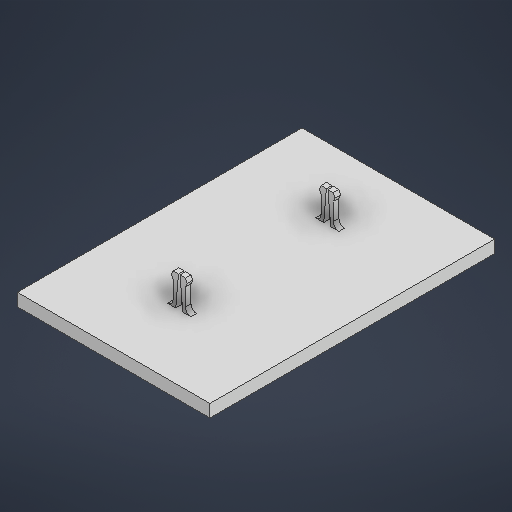
# Autodesk Inventor part: Bolt Slot Covers
Saved by Autodesk Inventor 2026.2 (Build 302298000, 298)
## iProperties
Created: 2026-05-27
Part Number: Bolt Slot Covers
Material: Generic
Document SubType Name: Modeling
Designer: mayhe
Density: 1 g/cm^3
Appearance: Default
Author: mayhe
Autodesk Inventor part; units mm, degrees
ref_plane "YZ Plane" through (0, 0, 0) normal (1, 0, 0) x (0, 1, 0)
ref_plane "XZ Plane" through (0, 0, 0) normal (0, 1, 0) x (-1, 0, 0)
ref_plane "XY Plane" through (0, 0, 0) normal (0, 0, 1) x (1, 0, 0)
sketch "Sketch1" plane through (0, 0, 0) normal (0, 1, 0) x (-1, 0, 0)
  line L0 (34.5, 51) -> (-34.5, 51)
  line L1 (-34.5, 51) -> (-34.5, -51)
  line L2 (-34.5, -51) -> (34.5, -51)
  line L3 (34.5, -51) -> (34.5, 51)
  line L4 (34.5, 51) -> (-34.5, -51) construction
  line L5 (-34.5, 51) -> (34.5, -51) construction
  point P0 (0, 0)
  dimension "d0" = 69
  dimension "d1" = 102
  constraints: 12 end point, 2 midpoint, 2 parallel, 1 horizontal, 1 perpendicular
  measures "d0" distance of L2.end L1.end
  measures "d1" distance of L1.end L0.end
extrude "Extrusion1" add sketch "Sketch1" along normal mid plane 5
sketch "Sketch3" plane through (0, 2.5, 0) normal (0, 1, 0) x (1, 0, 0)
  line L0 (0, 26.5) -> (0, -26.5)
  line L1 (-2.2, 27.5) -> (2.2, 27.5)
  line L2 (2.2, 27.5) -> (2.2, 25.5)
  line L3 (2.2, 25.5) -> (-2.2, 25.5)
  line L4 (-2.2, 25.5) -> (-2.2, 27.5)
  line L5 (-2.2, 27.5) -> (2.2, 25.5) construction
  line L6 (2.2, 27.5) -> (-2.2, 25.5) construction
  line L7 (-1.25, 27.5) -> (1.25, 27.5)
  line L8 (1.25, 27.5) -> (1.25, 25.5)
  line L9 (1.25, 25.5) -> (-1.25, 25.5)
  line L10 (-1.25, 25.5) -> (-1.25, 27.5)
  line L11 (-1.25, 27.5) -> (1.25, 25.5) construction
  line L12 (1.25, 27.5) -> (-1.25, 25.5) construction
  point P0 (0, 0)
  point P1 (1.25, 27.5)
  point P2 (-1.25, 25.5)
  point P3 (-1.25, 27.5)
  dimension "d13" = 53
  dimension "d14" = 4.4
  dimension "d15" = 2
  dimension "d18" = 2.5
  constraints: 26 end point, 5 midpoint, 4 parallel, 2 horizontal, 2 perpendicular, 1 point on line, 1 vertical
  measures "d13" distance of L0.start L0.end
  measures "d14" distance of L2.end L3.end
  measures "d15" distance between parallel lines of L3 L1
  measures "d18" distance of L8.end L9.end
extrude "Extrusion3" add sketch "Sketch3" along normal blind 11 contours L1 L2 L3 L8
sketch "Sketch4" plane through (2.2, 2.5, -27.5) normal (0, 0, -1) x (-1, 0, 0)
  line L0 (0, 0) -> (0, 11) projected
  line L1 (0, 11) -> (-0.6339, 9.6405)
  line L2 (0, 11) -> (1.5, 11) construction
  line L3 (-0.6339, 9.6405) -> (0, 8.2811)
  point P0 (2.2, -2.5)
  point P1 (0, 8.2811)
  dimension "d19" = 1.5
  dimension "d20" = 115
  dimension "d21" = 1.5
  constraints: 6 end point, 1 equal length, 1 horizontal
  measures "d19" distance of L0.end L1.end
  measures "d20" angle of L1 L2
  measures "d21" distance of L1.end L3.end
extrude "Extrusion4" add sketch "Sketch4" against normal up to surface (2 mm away)
fillet "Fillet1" radius 2 1 edges at (2.2, 2.5, -26.5)
draft "FaceDraft1" angle -5 pull direction (0, 1, 0) faces at (1.25, 6.1667, -26.8333) fixed edges at (1.25, 2.5, -26.5)
mirror "Mirror1" about plane through (0, 0, 0) normal (1, 0, 0) of "Extrusion4", "Extrusion3", "FaceDraft1", "Fillet1"
mirror "Mirror2" about plane through (0, 0, 0) normal (0, 0, 1) of "Extrusion4", "Extrusion3", "FaceDraft1", "Fillet1", "Mirror1"
chamfer "Chamfer2" distance 0.5 angle 45 4 edges at (0, -2.5, 51) (34.5, -2.5, 0) (-34.5, -2.5, 0) (0, -2.5, -51)
sketch "Sketch5" plane through (0, -2.5, 0) normal (0, -1, 0) x (1, 0, 0)
  line L0 (-43.2011, -30.2935) -> (-43.2011, 28.7129) construction
  line L1 (-43.2011, 28.7129) -> (40.8303, 28.7129) construction
  line L2 (40.8303, 28.7129) -> (40.8303, -30.2935) construction
  line L3 (40.8303, -30.2935) -> (-43.2011, -30.2935) construction
  spline S0 degree 2 poles (-3.5733, -17.3493) (-3.5733, -18.0112) (-3.8499, -18.9399) (-4.0475, -19.35) knots 0 0 0 1 2 2 2
  line L4 (-4.0475, -19.35) -> (-5.0652, -19.35)
  line L5 (-5.0652, -19.35) -> (-5.0652, -19.2907)
  spline S1 degree 2 poles (-5.0652, -19.2907) (-4.6897, -18.8905) (-4.2748, -17.8778) (-4.2748, -17.4085) knots 0 0 0 1 2 2 2
  spline S2 degree 2 poles (-4.2748, -17.4085) (-4.2748, -16.7367) (-4.833, -16.05) (-5.2924, -16.05) knots 0 0 0 1 2 2 2
  spline S3 degree 2 poles (-5.2924, -16.05) (-5.658, -16.05) (-6.1125, -16.4106) (-6.2261, -16.8009) knots 0 0 0 1 2 2 2
  spline S4 degree 2 poles (-6.2261, -16.8009) (-6.3051, -17.0825) (-6.4138, -17.5518) (-6.5027, -17.9025) knots 0 0 0 1 2 2 2
  spline S5 degree 2 poles (-6.5027, -17.9025) (-6.5867, -18.2187) (-6.8386, -18.7176) (-7.0412, -18.9103) knots 0 0 0 1 2 2 2
  spline S6 degree 2 poles (-7.0412, -18.9103) (-7.2437, -19.098) (-7.7871, -19.3055) (-8.1428, -19.3055) knots 0 0 0 1 2 2 2
  spline S7 degree 2 poles (-8.1428, -19.3055) (-8.8838, -19.3055) (-9.8866, -18.1495) (-9.8866, -17.2554) knots 0 0 0 1 2 2 2
  spline S8 degree 2 poles (-9.8866, -17.2554) (-9.8866, -16.7416) (-9.6841, -15.8327) (-9.4914, -15.4424) knots 0 0 0 1 2 2 2
  line L6 (-9.4914, -15.4424) -> (-8.5232, -15.4424)
  line L7 (-8.5232, -15.4424) -> (-8.5232, -15.5017)
  spline S9 degree 2 poles (-8.5232, -15.5017) (-8.79, -15.7931) (-9.1852, -16.7021) (-9.1852, -17.2011) knots 0 0 0 1 2 2 2
  spline S10 degree 2 poles (-9.1852, -17.2011) (-9.1852, -17.7642) (-8.6566, -18.4608) (-8.2268, -18.4608) knots 0 0 0 1 2 2 2
  spline S11 degree 2 poles (-8.2268, -18.4608) (-7.8415, -18.4608) (-7.382, -18.0507) (-7.2783, -17.6654) knots 0 0 0 1 2 2 2
  spline S12 degree 2 poles (-7.2783, -17.6654) (-7.2091, -17.4085) (-7.0313, -16.6626) (-6.9572, -16.4156) knots 0 0 0 1 2 2 2
  spline S13 degree 2 poles (-6.9572, -16.4156) (-6.7645, -15.7882) (-5.989, -15.2053) (-5.4209, -15.2053) knots 0 0 0 1 2 2 2
  spline S14 degree 2 poles (-5.4209, -15.2053) (-5.0602, -15.2053) (-4.3686, -15.4967) (-4.1266, -15.7586) knots 0 0 0 1 2 2 2
  spline S15 degree 2 poles (-4.1266, -15.7586) (-3.8598, -16.05) (-3.5733, -16.791) (-3.5733, -17.3493) knots 0 0 0 1 2 2 2
  line L8 (-3.682, -13.6541) -> (-3.682, -14.4248)
  line L9 (-3.682, -14.4248) -> (-10.0497, -14.4248)
  line L10 (-10.0497, -14.4248) -> (-10.0497, -13.6541)
  line L11 (-10.0497, -13.6541) -> (-3.682, -13.6541)
  spline S16 degree 2 poles (-5.9692, -8.7635) (-4.8132, -8.7635) (-3.5535, -9.875) (-3.5535, -10.8037) knots 0 0 0 1 2 2 2
  spline S17 degree 2 poles (-3.5535, -10.8037) (-3.5535, -11.7571) (-4.8527, -12.8489) (-5.9692, -12.8489) knots 0 0 0 1 2 2 2
  spline S18 degree 2 poles (-5.9692, -12.8489) (-7.1153, -12.8489) (-8.3849, -11.7226) (-8.3849, -10.8037) knots 0 0 0 1 2 2 2
  spline S19 degree 2 poles (-8.3849, -10.8037) (-8.3849, -9.875) (-7.1202, -8.7635) (-5.9692, -8.7635) knots 0 0 0 1 2 2 2
  spline S20 degree 2 poles (-5.9692, -9.5588) (-6.8584, -9.5588) (-7.7229, -10.206) (-7.7229, -10.8037) knots 0 0 0 1 2 2 2
  spline S21 degree 2 poles (-7.7229, -10.8037) (-7.7229, -11.4015) (-6.8584, -12.0535) (-5.9692, -12.0535) knots 0 0 0 1 2 2 2
  spline S22 degree 2 poles (-5.9692, -12.0535) (-5.1047, -12.0535) (-4.2155, -11.4015) (-4.2155, -10.8037) knots 0 0 0 1 2 2 2
  spline S23 degree 2 poles (-4.2155, -10.8037) (-4.2155, -10.2109) (-5.0899, -9.5588) (-5.9692, -9.5588) knots 0 0 0 1 2 2 2
  spline S24 degree 2 poles (-3.593, -6.5899) (-3.593, -7.2172) (-4.3093, -7.9237) (-5.0849, -7.9237) knots 0 0 0 1 2 2 2
  line L12 (-5.0849, -7.9237) -> (-7.6192, -7.9237)
  line L13 (-7.6192, -7.9237) -> (-7.6192, -8.4424)
  line L14 (-7.6192, -8.4424) -> (-8.2564, -8.4424)
  line L15 (-8.2564, -8.4424) -> (-8.2564, -7.9237)
  line L16 (-8.2564, -7.9237) -> (-9.5705, -7.9237)
  line L17 (-9.5705, -7.9237) -> (-9.5705, -7.153)
  line L18 (-9.5705, -7.153) -> (-8.2564, -7.153)
  line L19 (-8.2564, -7.153) -> (-8.2564, -5.7352)
  line L20 (-8.2564, -5.7352) -> (-7.6192, -5.7352)
  line L21 (-7.6192, -5.7352) -> (-7.6192, -7.153)
  line L22 (-7.6192, -7.153) -> (-5.4406, -7.153)
  spline S25 degree 2 poles (-5.4406, -7.153) (-5.0948, -7.153) (-4.7144, -7.1283) (-4.5514, -7.0443) knots 0 0 0 1 2 2 2
  spline S26 degree 2 poles (-4.5514, -7.0443) (-4.4081, -6.9752) (-4.2649, -6.664) (-4.2649, -6.3972) knots 0 0 0 1 2 2 2
  spline S27 degree 2 poles (-4.2649, -6.3972) (-4.2649, -6.2095) (-4.3785, -5.8587) (-4.4131, -5.7797) knots 0 0 0 1 2 2 2
  line L23 (-4.4131, -5.7797) -> (-4.4131, -5.7352)
  line L24 (-4.4131, -5.7352) -> (-3.7215, -5.7352)
  spline S28 degree 2 poles (-3.7215, -5.7352) (-3.6622, -5.9526) (-3.593, -6.3972) (-3.593, -6.5899) knots 0 0 0 1 2 2 2
  spline S29 degree 2 poles (-3.5733, -0.1085) (-3.5733, -0.7013) (-3.9734, -1.7042) (-4.3736, -2.0697) knots 0 0 0 1 2 2 2
  spline S30 degree 2 poles (-4.3736, -2.0697) (-4.7688, -2.4353) (-5.9544, -2.8354) (-6.725, -2.8354) knots 0 0 0 1 2 2 2
  spline S31 degree 2 poles (-6.725, -2.8354) (-7.4907, -2.8354) (-8.6269, -2.4452) (-9.0468, -2.0747) knots 0 0 0 1 2 2 2
  spline S32 degree 2 poles (-9.0468, -2.0747) (-9.4569, -1.7091) (-9.8866, -0.7112) (-9.8866, -0.0937) knots 0 0 0 1 2 2 2
  spline S33 degree 2 poles (-9.8866, -0.0937) (-9.8866, 0.2126) (-9.7977, 0.751) (-9.7286, 0.9783) knots 0 0 0 1 2 2 2
  spline S34 degree 2 poles (-9.7286, 0.9783) (-9.6643, 1.1759) (-9.4816, 1.5859) (-9.3729, 1.7884) knots 0 0 0 1 2 2 2
  line L25 (-9.3729, 1.7884) -> (-8.3948, 1.7884)
  line L26 (-8.3948, 1.7884) -> (-8.3948, 1.7242)
  spline S35 degree 2 poles (-8.3948, 1.7242) (-8.4936, 1.6155) (-8.7702, 1.2796) (-8.9036, 1.0375) knots 0 0 0 1 2 2 2
  spline S36 degree 2 poles (-8.9036, 1.0375) (-9.032, 0.8054) (-9.195, 0.257) (-9.195, -0.0987) knots 0 0 0 1 2 2 2
  spline S37 degree 2 poles (-9.195, -0.0987) (-9.195, -0.4889) (-8.8739, -1.1855) (-8.5677, -1.4473) knots 0 0 0 1 2 2 2
  spline S38 degree 2 poles (-8.5677, -1.4473) (-8.2564, -1.7042) (-7.3129, -1.9907) (-6.725, -1.9907) knots 0 0 0 1 2 2 2
  spline S39 degree 2 poles (-6.725, -1.9907) (-6.0976, -1.9907) (-5.1936, -1.6894) (-4.8824, -1.4275) knots 0 0 0 1 2 2 2
  spline S40 degree 2 poles (-4.8824, -1.4275) (-4.581, -1.1706) (-4.2748, -0.484) (-4.2748, -0.0987) knots 0 0 0 1 2 2 2
  spline S41 degree 2 poles (-4.2748, -0.0987) (-4.2748, 0.2521) (-4.4477, 0.8498) (-4.5761, 1.082) knots 0 0 0 1 2 2 2
  spline S42 degree 2 poles (-4.5761, 1.082) (-4.7045, 1.3043) (-4.9713, 1.6353) (-5.0652, 1.7292) knots 0 0 0 1 2 2 2
  line L27 (-5.0652, 1.7292) -> (-5.0652, 1.7884)
  line L28 (-5.0652, 1.7884) -> (-4.0969, 1.7884)
  spline S43 degree 2 poles (-4.0969, 1.7884) (-4.0031, 1.5859) (-3.8302, 1.2302) (-3.7511, 0.9783) knots 0 0 0 1 2 2 2
  spline S44 degree 2 poles (-3.7511, 0.9783) (-3.6622, 0.7115) (-3.5733, 0.257) (-3.5733, -0.1085) knots 0 0 0 1 2 2 2
  spline S45 degree 2 poles (-5.9692, 6.2443) (-4.8132, 6.2443) (-3.5535, 5.1328) (-3.5535, 4.2041) knots 0 0 0 1 2 2 2
  spline S46 degree 2 poles (-3.5535, 4.2041) (-3.5535, 3.2507) (-4.8527, 2.1589) (-5.9692, 2.1589) knots 0 0 0 1 2 2 2
  spline S47 degree 2 poles (-5.9692, 2.1589) (-7.1153, 2.1589) (-8.3849, 3.2853) (-8.3849, 4.2041) knots 0 0 0 1 2 2 2
  spline S48 degree 2 poles (-8.3849, 4.2041) (-8.3849, 5.1328) (-7.1202, 6.2443) (-5.9692, 6.2443) knots 0 0 0 1 2 2 2
  spline S49 degree 2 poles (-5.9692, 5.449) (-6.8584, 5.449) (-7.7229, 4.8019) (-7.7229, 4.2041) knots 0 0 0 1 2 2 2
  spline S50 degree 2 poles (-7.7229, 4.2041) (-7.7229, 3.6064) (-6.8584, 2.9543) (-5.9692, 2.9543) knots 0 0 0 1 2 2 2
  spline S51 degree 2 poles (-5.9692, 2.9543) (-5.1047, 2.9543) (-4.2155, 3.6064) (-4.2155, 4.2041) knots 0 0 0 1 2 2 2
  spline S52 degree 2 poles (-4.2155, 4.2041) (-4.2155, 4.7969) (-5.0899, 5.449) (-5.9692, 5.449) knots 0 0 0 1 2 2 2
  line L29 (-8.2564, 10.6262) -> (-3.682, 8.9021)
  line L30 (-3.682, 8.9021) -> (-3.682, 8.2105)
  line L31 (-3.682, 8.2105) -> (-8.2564, 6.5012)
  line L32 (-8.2564, 6.5012) -> (-8.2564, 7.3361)
  line L33 (-8.2564, 7.3361) -> (-4.7342, 8.5859)
  line L34 (-4.7342, 8.5859) -> (-8.2564, 9.8259)
  line L35 (-8.2564, 9.8259) -> (-8.2564, 10.6262)
  spline S53 degree 2 poles (-3.5782, 13.195) (-3.5782, 12.0983) (-4.8083, 10.8929) (-5.9445, 10.8929) knots 0 0 0 1 2 2 2
  spline S54 degree 2 poles (-5.9445, 10.8929) (-7.0609, 10.8929) (-8.3849, 12.0637) (-8.3849, 13.0072) knots 0 0 0 1 2 2 2
  spline S55 degree 2 poles (-8.3849, 13.0072) (-8.3849, 13.4321) (-8.1379, 14.0891) (-7.876, 14.3312) knots 0 0 0 1 2 2 2
  spline S56 degree 2 poles (-7.876, 14.3312) (-7.6142, 14.5782) (-6.8584, 14.84) (-6.3101, 14.84) knots 0 0 0 1 2 2 2
  line L36 (-6.3101, 14.84) -> (-5.8902, 14.84)
  line L37 (-5.8902, 14.84) -> (-5.8902, 11.6734)
  spline S57 degree 2 poles (-5.8902, 11.6734) (-5.0948, 11.6734) (-4.2501, 12.4737) (-4.2501, 13.1851) knots 0 0 0 1 2 2 2
  spline S58 degree 2 poles (-4.2501, 13.1851) (-4.2501, 13.437) (-4.3637, 13.9261) (-4.4526, 14.1237) knots 0 0 0 1 2 2 2
  spline S59 degree 2 poles (-4.4526, 14.1237) (-4.5514, 14.3312) (-4.7243, 14.6177) (-4.8033, 14.7116) knots 0 0 0 1 2 2 2
  line L38 (-4.8033, 14.7116) -> (-4.8033, 14.756)
  line L39 (-4.8033, 14.756) -> (-3.9635, 14.756)
  spline S60 degree 2 poles (-3.9635, 14.756) (-3.9092, 14.6226) (-3.7511, 14.2176) (-3.7067, 14.0595) knots 0 0 0 1 2 2 2
  spline S61 degree 2 poles (-3.7067, 14.0595) (-3.6424, 13.8372) (-3.5782, 13.4716) (-3.5782, 13.195) knots 0 0 0 1 2 2 2
  spline S62 degree 2 poles (-6.478, 14.0891) (-6.7892, 14.0792) (-7.2437, 13.9508) (-7.3969, 13.8273) knots 0 0 0 1 2 2 2
  spline S63 degree 2 poles (-7.3969, 13.8273) (-7.5698, 13.6939) (-7.7525, 13.274) (-7.7525, 12.9628) knots 0 0 0 1 2 2 2
  spline S64 degree 2 poles (-7.7525, 12.9628) (-7.7525, 12.6565) (-7.5698, 12.2267) (-7.3919, 12.0489) knots 0 0 0 1 2 2 2
  spline S65 degree 2 poles (-7.3919, 12.0489) (-7.2091, 11.876) (-6.7695, 11.6981) (-6.478, 11.6734) knots 0 0 0 1 2 2 2
  line L40 (-6.478, 11.6734) -> (-6.478, 14.0891)
  line L41 (-7.4314, 18.0461) -> (-7.4314, 18.0066)
  spline S66 degree 2 poles (-7.4314, 18.0066) (-7.4561, 17.9176) (-7.466, 17.725) (-7.466, 17.5916) knots 0 0 0 1 2 2 2
  spline S67 degree 2 poles (-7.466, 17.5916) (-7.466, 17.2804) (-7.1943, 16.6678) (-6.9276, 16.3912) knots 0 0 0 1 2 2 2
  line L42 (-6.9276, 16.3912) -> (-3.682, 16.3912)
  line L43 (-3.682, 16.3912) -> (-3.682, 15.6205)
  line L44 (-3.682, 15.6205) -> (-8.2564, 15.6205)
  line L45 (-8.2564, 15.6205) -> (-8.2564, 16.3912)
  line L46 (-8.2564, 16.3912) -> (-7.5747, 16.3912)
  spline S68 degree 2 poles (-7.5747, 16.3912) (-7.9502, 16.8111) (-8.2564, 17.4385) (-8.2564, 17.7349) knots 0 0 0 1 2 2 2
  spline S69 degree 2 poles (-8.2564, 17.7349) (-8.2564, 17.8534) (-8.2466, 17.972) (-8.2317, 18.0461) knots 0 0 0 1 2 2 2
  line L47 (-8.2317, 18.0461) -> (-7.4314, 18.0461)
  spline S70 degree 2 poles (4.4184, -15.8672) (4.8581, -15.8672) (5.609, -16.1488) (5.8856, -16.4057) knots 0 0 0 1 2 2 2
  spline S71 degree 2 poles (5.8856, -16.4057) (6.1623, -16.6626) (6.4834, -17.4283) (6.4834, -17.9025) knots 0 0 0 1 2 2 2
  spline S72 degree 2 poles (6.4834, -17.9025) (6.4834, -18.3373) (6.2907, -19.1869) (6.1376, -19.4982) knots 0 0 0 1 2 2 2
  line L48 (6.1376, -19.4982) -> (5.2731, -19.4982)
  line L49 (5.2731, -19.4982) -> (5.2731, -19.4389)
  spline S73 degree 2 poles (5.2731, -19.4389) (5.3422, -19.345) (5.5201, -18.9943) (5.5991, -18.7819) knots 0 0 0 1 2 2 2
  spline S74 degree 2 poles (5.5991, -18.7819) (5.6831, -18.5398) (5.777, -18.1397) (5.777, -17.8877) knots 0 0 0 1 2 2 2
  spline S75 degree 2 poles (5.777, -17.8877) (5.777, -17.6407) (5.5991, -17.1764) (5.4065, -17.0084) knots 0 0 0 1 2 2 2
  spline S76 degree 2 poles (5.4065, -17.0084) (5.2237, -16.8552) (4.7396, -16.6972) (4.4135, -16.6972) knots 0 0 0 1 2 2 2
  spline S77 degree 2 poles (4.4135, -16.6972) (4.0875, -16.6972) (3.6725, -16.875) (3.5342, -17.043) knots 0 0 0 1 2 2 2
  spline S78 degree 2 poles (3.5342, -17.043) (3.381, -17.2159) (3.2526, -17.7296) (3.2526, -18.0409) knots 0 0 0 1 2 2 2
  spline S79 degree 2 poles (3.2526, -18.0409) (3.2526, -18.3768) (3.3563, -19.0437) (3.4008, -19.2462) knots 0 0 0 1 2 2 2
  line L50 (3.4008, -19.2462) -> (0.2589, -19.2462)
  line L51 (0.2589, -19.2462) -> (0.2589, -15.9018)
  line L52 (0.2589, -15.9018) -> (0.9752, -15.9018)
  line L53 (0.9752, -15.9018) -> (0.9752, -18.4608)
  line L54 (0.9752, -18.4608) -> (2.6005, -18.4608)
  spline S80 degree 2 poles (2.6005, -18.4608) (2.5808, -18.3126) (2.5659, -18.026) (2.5659, -17.9075) knots 0 0 0 1 2 2 2
  spline S81 degree 2 poles (2.5659, -17.9075) (2.5659, -17.4382) (2.7191, -16.791) (2.9463, -16.4946) knots 0 0 0 1 2 2 2
  spline S82 degree 2 poles (2.9463, -16.4946) (3.1736, -16.1933) (3.8652, -15.8672) (4.4184, -15.8672) knots 0 0 0 1 2 2 2
  line L55 (-0.0128, -12.4537) -> (7.6789, -14.8397)
  line L56 (7.6789, -14.8397) -> (7.6789, -15.5313)
  line L57 (7.6789, -15.5313) -> (-0.0128, -13.1552)
  line L58 (-0.0128, -13.1552) -> (-0.0128, -12.4537)
  line L59 (6.3549, -8.0225) -> (6.3549, -11.7818)
  line L60 (6.3549, -11.7818) -> (5.4904, -11.7818)
  spline S83 degree 2 poles (5.4904, -11.7818) (5.1101, -11.3768) (4.4036, -10.6555) (4.0232, -10.3097) knots 0 0 0 1 2 2 2
  spline S84 degree 2 poles (4.0232, -10.3097) (3.2575, -9.6132) (2.3387, -9.1043) (1.8496, -9.1043) knots 0 0 0 1 2 2 2
  spline S85 degree 2 poles (1.8496, -9.1043) (1.5928, -9.1043) (1.2074, -9.2624) (1.0839, -9.4057) knots 0 0 0 1 2 2 2
  spline S86 degree 2 poles (1.0839, -9.4057) (0.9604, -9.5489) (0.8369, -9.9244) (0.8369, -10.1516) knots 0 0 0 1 2 2 2
  spline S87 degree 2 poles (0.8369, -10.1516) (0.8369, -10.369) (0.9456, -10.8136) (1.0296, -11.0161) knots 0 0 0 1 2 2 2
  spline S88 degree 2 poles (1.0296, -11.0161) (1.0987, -11.189) (1.2963, -11.5101) (1.3655, -11.6089) knots 0 0 0 1 2 2 2
  line L61 (1.3655, -11.6089) -> (1.3655, -11.6534)
  line L62 (1.3655, -11.6534) -> (0.4961, -11.6534)
  spline S89 degree 2 poles (0.4961, -11.6534) (0.3726, -11.4015) (0.1305, -10.4974) (0.1305, -10.0923) knots 0 0 0 1 2 2 2
  spline S90 degree 2 poles (0.1305, -10.0923) (0.1305, -9.2377) (1.0345, -8.2744) (1.8052, -8.2744) knots 0 0 0 1 2 2 2
  spline S91 degree 2 poles (1.8052, -8.2744) (2.1658, -8.2744) (2.7685, -8.4424) (3.0254, -8.5906) knots 0 0 0 1 2 2 2
  spline S92 degree 2 poles (3.0254, -8.5906) (3.2921, -8.7388) (3.8158, -9.1686) (4.0677, -9.4057) knots 0 0 0 1 2 2 2
  spline S93 degree 2 poles (4.0677, -9.4057) (4.4876, -9.791) (5.3867, -10.7345) (5.6485, -11.0161) knots 0 0 0 1 2 2 2
  line L63 (5.6485, -11.0161) -> (5.6485, -8.0225)
  line L64 (5.6485, -8.0225) -> (6.3549, -8.0225)
  spline S94 degree 2 poles (6.4933, -5.3647) (6.4933, -5.8192) (6.2216, -6.5652) (5.9696, -6.827) knots 0 0 0 1 2 2 2
  spline S95 degree 2 poles (5.9696, -6.827) (5.7226, -7.0839) (5.0508, -7.3506) (4.6704, -7.3506) knots 0 0 0 1 2 2 2
  spline S96 degree 2 poles (4.6704, -7.3506) (4.1764, -7.3506) (3.3465, -6.822) (3.0995, -6.3182) knots 0 0 0 1 2 2 2
  line L65 (3.0995, -6.3182) -> (3.0748, -6.3182)
  spline S97 degree 2 poles (3.0748, -6.3182) (2.8129, -6.7677) (2.1905, -7.2024) (1.7261, -7.2024) knots 0 0 0 1 2 2 2
  spline S98 degree 2 poles (1.7261, -7.2024) (1.0395, -7.2024) (0.1206, -6.165) (0.1206, -5.3647) knots 0 0 0 1 2 2 2
  spline S99 degree 2 poles (0.1206, -5.3647) (0.1206, -4.5348) (0.9901, -3.532) (1.6718, -3.532) knots 0 0 0 1 2 2 2
  spline S100 degree 2 poles (1.6718, -3.532) (2.0818, -3.532) (2.8821, -4.0112) (3.1093, -4.4607) knots 0 0 0 1 2 2 2
  line L66 (3.1093, -4.4607) -> (3.134, -4.4607)
  spline S101 degree 2 poles (3.134, -4.4607) (3.381, -3.9272) (4.0924, -3.3788) (4.6556, -3.3788) knots 0 0 0 1 2 2 2
  spline S102 degree 2 poles (4.6556, -3.3788) (5.4361, -3.3788) (6.4933, -4.515) (6.4933, -5.3647) knots 0 0 0 1 2 2 2
  spline S103 degree 2 poles (4.7346, -4.2186) (4.3592, -4.2186) (3.9146, -4.515) (3.6873, -4.935) knots 0 0 0 1 2 2 2
  spline S104 degree 2 poles (3.6873, -4.935) (3.6083, -5.0733) (3.4255, -5.5376) (3.3069, -5.8291) knots 0 0 0 1 2 2 2
  spline S105 degree 2 poles (3.3069, -5.8291) (3.5292, -6.165) (4.1912, -6.5256) (4.6111, -6.5256) knots 0 0 0 1 2 2 2
  spline S106 degree 2 poles (4.6111, -6.5256) (5.1644, -6.5256) (5.8856, -5.8587) (5.8856, -5.3549) knots 0 0 0 1 2 2 2
  spline S107 degree 2 poles (5.8856, -5.3549) (5.8856, -4.8411) (5.2681, -4.2186) (4.7346, -4.2186) knots 0 0 0 1 2 2 2
  spline S108 degree 2 poles (1.6817, -4.3323) (1.2716, -4.3323) (0.7233, -4.8806) (0.7233, -5.3697) knots 0 0 0 1 2 2 2
  spline S109 degree 2 poles (0.7233, -5.3697) (0.7233, -5.8143) (1.2124, -6.3824) (1.6323, -6.3824) knots 0 0 0 1 2 2 2
  spline S110 degree 2 poles (1.6323, -6.3824) (1.9336, -6.3824) (2.3535, -6.0909) (2.5215, -5.7995) knots 0 0 0 1 2 2 2
  spline S111 degree 2 poles (2.5215, -5.7995) (2.5906, -5.676) (2.8327, -5.1523) (2.9019, -4.9399) knots 0 0 0 1 2 2 2
  spline S112 degree 2 poles (2.9019, -4.9399) (2.6302, -4.5842) (2.0522, -4.3323) (1.6817, -4.3323) knots 0 0 0 1 2 2 2
  line L67 (-0.0128, -0.0987) -> (7.6789, -2.4847)
  line L68 (7.6789, -2.4847) -> (7.6789, -3.1763)
  line L69 (7.6789, -3.1763) -> (-0.0128, -0.8001)
  line L70 (-0.0128, -0.8001) -> (-0.0128, -0.0987)
  line L71 (6.3549, 4.3325) -> (6.3549, 0.5732)
  line L72 (6.3549, 0.5732) -> (5.4904, 0.5732)
  spline S113 degree 2 poles (5.4904, 0.5732) (5.1101, 0.9783) (4.4036, 1.6995) (4.0232, 2.0453) knots 0 0 0 1 2 2 2
  spline S114 degree 2 poles (4.0232, 2.0453) (3.2575, 2.7419) (2.3387, 3.2507) (1.8496, 3.2507) knots 0 0 0 1 2 2 2
  spline S115 degree 2 poles (1.8496, 3.2507) (1.5928, 3.2507) (1.2074, 3.0926) (1.0839, 2.9493) knots 0 0 0 1 2 2 2
  spline S116 degree 2 poles (1.0839, 2.9493) (0.9604, 2.8061) (0.8369, 2.4306) (0.8369, 2.2034) knots 0 0 0 1 2 2 2
  spline S117 degree 2 poles (0.8369, 2.2034) (0.8369, 1.986) (0.9456, 1.5414) (1.0296, 1.3389) knots 0 0 0 1 2 2 2
  spline S118 degree 2 poles (1.0296, 1.3389) (1.0987, 1.166) (1.2963, 0.8449) (1.3655, 0.7461) knots 0 0 0 1 2 2 2
  line L73 (1.3655, 0.7461) -> (1.3655, 0.7016)
  line L74 (1.3655, 0.7016) -> (0.4961, 0.7016)
  spline S119 degree 2 poles (0.4961, 0.7016) (0.3726, 0.9536) (0.1305, 1.8576) (0.1305, 2.2627) knots 0 0 0 1 2 2 2
  spline S120 degree 2 poles (0.1305, 2.2627) (0.1305, 3.1173) (1.0345, 4.0806) (1.8052, 4.0806) knots 0 0 0 1 2 2 2
  spline S121 degree 2 poles (1.8052, 4.0806) (2.1658, 4.0806) (2.7685, 3.9126) (3.0254, 3.7644) knots 0 0 0 1 2 2 2
  spline S122 degree 2 poles (3.0254, 3.7644) (3.2921, 3.6162) (3.8158, 3.1865) (4.0677, 2.9493) knots 0 0 0 1 2 2 2
  spline S123 degree 2 poles (4.0677, 2.9493) (4.4876, 2.564) (5.3867, 1.6205) (5.6485, 1.3389) knots 0 0 0 1 2 2 2
  line L75 (5.6485, 1.3389) -> (5.6485, 4.3325)
  line L76 (5.6485, 4.3325) -> (6.3549, 4.3325)
  spline S124 degree 2 poles (3.3069, 8.9416) (4.947, 8.9416) (6.4834, 7.9882) (6.4834, 6.9952) knots 0 0 0 1 2 2 2
  spline S125 degree 2 poles (6.4834, 6.9952) (6.4834, 5.9875) (4.9174, 5.0439) (3.3119, 5.0439) knots 0 0 0 1 2 2 2
  spline S126 degree 2 poles (3.3119, 5.0439) (1.6619, 5.0439) (0.1354, 5.9973) (0.1354, 6.9952) knots 0 0 0 1 2 2 2
  spline S127 degree 2 poles (0.1354, 6.9952) (0.1354, 7.9981) (1.7163, 8.9416) (3.3069, 8.9416) knots 0 0 0 1 2 2 2
  spline S128 degree 2 poles (5.1644, 7.8943) (4.8631, 8.0129) (3.9343, 8.1117) (3.3069, 8.1117) knots 0 0 0 1 2 2 2
  spline S129 degree 2 poles (3.3069, 8.1117) (2.6796, 8.1117) (1.7558, 8.0129) (1.4445, 7.8894) knots 0 0 0 1 2 2 2
  spline S130 degree 2 poles (1.4445, 7.8894) (1.1333, 7.7659) (0.8122, 7.3361) (0.8122, 6.9952) knots 0 0 0 1 2 2 2
  spline S131 degree 2 poles (0.8122, 6.9952) (0.8122, 6.6544) (1.1333, 6.2147) (1.4544, 6.0863) knots 0 0 0 1 2 2 2
  spline S132 degree 2 poles (1.4544, 6.0863) (1.7657, 5.9628) (2.7141, 5.8738) (3.3119, 5.8738) knots 0 0 0 1 2 2 2
  spline S133 degree 2 poles (3.3119, 5.8738) (3.9541, 5.8738) (4.8137, 5.9529) (5.1496, 6.0813) knots 0 0 0 1 2 2 2
  spline S134 degree 2 poles (5.1496, 6.0813) (5.4657, 6.1999) (5.8066, 6.6395) (5.8066, 6.9952) knots 0 0 0 1 2 2 2
  spline S135 degree 2 poles (5.8066, 6.9952) (5.8066, 7.3311) (5.4855, 7.7708) (5.1644, 7.8943) knots 0 0 0 1 2 2 2
  line L77 (6.3549, 13.4815) -> (6.3549, 9.7221)
  line L78 (6.3549, 9.7221) -> (5.4904, 9.7221)
  spline S136 degree 2 poles (5.4904, 9.7221) (5.1101, 10.1272) (4.4036, 10.8485) (4.0232, 11.1943) knots 0 0 0 1 2 2 2
  spline S137 degree 2 poles (4.0232, 11.1943) (3.2575, 11.8908) (2.3387, 12.3996) (1.8496, 12.3996) knots 0 0 0 1 2 2 2
  spline S138 degree 2 poles (1.8496, 12.3996) (1.5928, 12.3996) (1.2074, 12.2415) (1.0839, 12.0983) knots 0 0 0 1 2 2 2
  spline S139 degree 2 poles (1.0839, 12.0983) (0.9604, 11.955) (0.8369, 11.5796) (0.8369, 11.3523) knots 0 0 0 1 2 2 2
  spline S140 degree 2 poles (0.8369, 11.3523) (0.8369, 11.135) (0.9456, 10.6904) (1.0296, 10.4878) knots 0 0 0 1 2 2 2
  spline S141 degree 2 poles (1.0296, 10.4878) (1.0987, 10.3149) (1.2963, 9.9938) (1.3655, 9.895) knots 0 0 0 1 2 2 2
  line L79 (1.3655, 9.895) -> (1.3655, 9.8506)
  line L80 (1.3655, 9.8506) -> (0.4961, 9.8506)
  spline S142 degree 2 poles (0.4961, 9.8506) (0.3726, 10.1025) (0.1305, 11.0065) (0.1305, 11.4116) knots 0 0 0 1 2 2 2
  spline S143 degree 2 poles (0.1305, 11.4116) (0.1305, 12.2662) (1.0345, 13.2295) (1.8052, 13.2295) knots 0 0 0 1 2 2 2
  spline S144 degree 2 poles (1.8052, 13.2295) (2.1658, 13.2295) (2.7685, 13.0616) (3.0254, 12.9134) knots 0 0 0 1 2 2 2
  spline S145 degree 2 poles (3.0254, 12.9134) (3.2921, 12.7652) (3.8158, 12.3354) (4.0677, 12.0983) knots 0 0 0 1 2 2 2
  spline S146 degree 2 poles (4.0677, 12.0983) (4.4876, 11.713) (5.3867, 10.7694) (5.6485, 10.4878) knots 0 0 0 1 2 2 2
  line L81 (5.6485, 10.4878) -> (5.6485, 13.4815)
  line L82 (5.6485, 13.4815) -> (6.3549, 13.4815)
  spline S147 degree 2 poles (4.3789, 18.1498) (4.8482, 18.1498) (5.6436, 17.8386) (5.9103, 17.5768) knots 0 0 0 1 2 2 2
  spline S148 degree 2 poles (5.9103, 17.5768) (6.1919, 17.3051) (6.4834, 16.6234) (6.4834, 16.2133) knots 0 0 0 1 2 2 2
  spline S149 degree 2 poles (6.4834, 16.2133) (6.4834, 15.8033) (6.2067, 15.1265) (5.9301, 14.8696) knots 0 0 0 1 2 2 2
  spline S150 degree 2 poles (5.9301, 14.8696) (5.5991, 14.5535) (4.4876, 14.1978) (3.6774, 14.1978) knots 0 0 0 1 2 2 2
  spline S151 degree 2 poles (3.6774, 14.1978) (2.8821, 14.1978) (1.6026, 14.5238) (1.1284, 14.8647) knots 0 0 0 1 2 2 2
  spline S152 degree 2 poles (1.1284, 14.8647) (0.664, 15.1957) (0.1453, 16.243) (0.1453, 16.9296) knots 0 0 0 1 2 2 2
  spline S153 degree 2 poles (0.1453, 16.9296) (0.1453, 17.1322) (0.1848, 17.4879) (0.2293, 17.6212) knots 0 0 0 1 2 2 2
  line L83 (0.2293, 17.6212) -> (1.0148, 17.6212)
  line L84 (1.0148, 17.6212) -> (1.0148, 17.5867)
  spline S154 degree 2 poles (1.0148, 17.5867) (0.9555, 17.473) (0.8517, 17.0581) (0.8517, 16.821) knots 0 0 0 1 2 2 2
  spline S155 degree 2 poles (0.8517, 16.821) (0.8517, 16.0602) (1.8793, 15.1265) (2.887, 15.0376) knots 0 0 0 1 2 2 2
  spline S156 degree 2 poles (2.887, 15.0376) (2.6845, 15.3291) (2.4622, 15.9416) (2.4622, 16.3072) knots 0 0 0 1 2 2 2
  spline S157 degree 2 poles (2.4622, 16.3072) (2.4622, 16.6629) (2.6055, 17.1964) (2.8228, 17.4879) knots 0 0 0 1 2 2 2
  spline S158 degree 2 poles (2.8228, 17.4879) (3.0748, 17.8238) (3.8553, 18.1498) (4.3789, 18.1498) knots 0 0 0 1 2 2 2
  spline S159 degree 2 poles (4.4135, 17.3199) (4.0381, 17.3199) (3.5292, 17.1223) (3.3514, 16.9049) knots 0 0 0 1 2 2 2
  spline S160 degree 2 poles (3.3514, 16.9049) (3.223, 16.7419) (3.139, 16.3368) (3.139, 16.1244) knots 0 0 0 1 2 2 2
  spline S161 degree 2 poles (3.139, 16.1244) (3.139, 15.8379) (3.3119, 15.2994) (3.4749, 15.0376) knots 0 0 0 1 2 2 2
  spline S162 degree 2 poles (3.4749, 15.0376) (3.5638, 15.0327) (3.7318, 15.0228) (3.8602, 15.0228) knots 0 0 0 1 2 2 2
  spline S163 degree 2 poles (3.8602, 15.0228) (4.4925, 15.0228) (5.2681, 15.2698) (5.4707, 15.4575) knots 0 0 0 1 2 2 2
  spline S164 degree 2 poles (5.4707, 15.4575) (5.6633, 15.6304) (5.8165, 16.0058) (5.8165, 16.2183) knots 0 0 0 1 2 2 2
  spline S165 degree 2 poles (5.8165, 16.2183) (5.8165, 16.7123) (5.115, 17.3199) (4.4135, 17.3199) knots 0 0 0 1 2 2 2
  point P0 (0, 0)
  dimension "d0" = 69
  dimension "d1" = 102
  constraints: 2 other
extrude "Extrusion5" cut sketch "Sketch5" against normal blind 1
body "Solid1"
